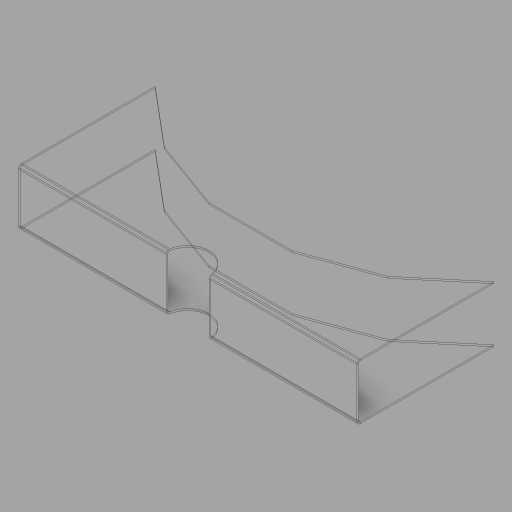
# Autodesk Inventor part: Halteblech
Saved by Autodesk Inventor 2023.2 (Build 272271000, 271)
## iProperties
Created: 2023-02-02
Part Number: Halteblech
Material: Generisch
Document SubType Name: Blech
Designer: Raoul Messerli
Density: 1 g/cm^3
Sheet Metal Rule: 3mm
Appearance: Vorgabe
Author: Raoul Messerli
Autodesk Inventor part; units mm, degrees
ref_plane "YZ Plane" through (0, 0, 0) normal (1, 0, 0) x (0, 1, 0)
ref_plane "XZ Plane" through (0, 0, 0) normal (0, 1, 0) x (-1, 0, 0)
ref_plane "XY Plane" through (0, 0, 0) normal (0, 0, 1) x (1, 0, 0)
sketch "Skizze1" plane through (0, 0, 0) normal (0, 0, 1) x (1, 0, 0)
  line L0 (300, -50) -> (-300, -50)
  line L1 (-300, -50) -> (-300, 50)
  line L2 (-300, 50) -> (300, 50)
  line L3 (300, 50) -> (300, -50)
  line L4 (300, -50) -> (-300, 50) construction
  line L5 (-300, -50) -> (300, 50) construction
  point P0 (0, 0)
  dimension "d0" = 600
  dimension "d1" = 100
  measures "d0" distance of L1.end L2.end
  measures "d1" distance of L0.end L1.end
extrude "Grobblech1" add sketch "Skizze1" along normal blind 3
sketch "Skizze2" plane through (300, 47, 3) normal (0, 1, 0) x (-1, 0, 0)
  line L0 (600, 0) -> (0, 0)
  line L1 (0, 0) -> (0, -250)
  line L2 (0, -250) -> (600, -250)
  line L3 (600, -250) -> (600, 0)
  constraints: 6 end point, 1 horizontal, 1 perpendicular, 1 vertical
edge flange "Lasche1" height 250 angle 90 thickness 3 bend radius 3 thickness toward (0, 1, 0) relief straight relief width 3 relief depth 1.5 edges at (0, 50, 0) wall of the first edge with corners at (-300, 47, 3) (300, 47, 3) (300, 47, -247) (-300, 47, -247)
bend "Biegung1"
corner "Ecke1"
sketch "Skizze3" plane through (-300, -47, 3) normal (0, -1, 0) x (1, 0, 0)
  line L0 (600, 0) -> (0, 0)
  line L1 (0, 0) -> (0, -250)
  line L2 (0, -250) -> (600, -250)
  line L3 (600, -250) -> (600, 0)
  constraints: 6 end point, 1 horizontal, 1 perpendicular, 1 vertical
edge flange "Lasche2" height 250 angle 90 thickness 3 bend radius 3 thickness toward (0, -1, 0) relief straight relief width 3 relief depth 1.5 edges at (0, -50, 0) wall of the first edge with corners at (300, -47, 3) (-300, -47, 3) (-300, -47, -247) (300, -47, -247)
bend "Biegung2"
corner "Ecke2"
sketch "Skizze4" plane through (0, 0, 0) normal (0, 1, 0) x (-1, 0, 0)
  line L0 (300, 3) -> (-300, 3) projected
  circle A0 centre (0, 3) radius 38.05
  point P0 (0, 0)
  dimension "d23" = 76.1
  constraints: 1 centre point, 1 midpoint
  measures "d23" diameter of A0
extrude "Extrusion1" cut sketch "Skizze4" along normal through all both and the other way through all
sketch "Skizze5" plane through (0, 0, 0) normal (0, 1, 0) x (-1, 0, 0)
  line L0 (-300, -3) -> (-300, -247) projected
  line L1 (-300, -239.3955) -> (-198.2712, -154.035)
  line L2 (-198.2712, -154.035) -> (-73.4825, -108.6156)
  line L3 (-73.4825, -108.6156) -> (73.4825, -108.6156)
  line L4 (73.4825, -108.6156) -> (198.2712, -154.035)
  line L5 (198.2712, -154.035) -> (300, -239.3955)
  line L6 (300, -3) -> (300, -247) projected
  line L7 (-300, -239.3955) -> (-300, -247)
  line L8 (-300, -247) -> (300, -247)
  line L9 (300, -247) -> (300, -239.3955)
  point P0 (0, 0)
  dimension "d26" = 160
  dimension "d27" = 160
  dimension "d28" = 160
  dimension "d29" = 160
  constraints: 16 end point, 3 equal length, 2 point on line, 1 collinear, 1 perpendicular
  measures "d26" angle of L3 L4
  measures "d27" angle of L5 L4
  measures "d28" angle of L3 L2
  measures "d29" angle of L1 L2
extrude "Extrusion2" cut sketch "Skizze5" along normal through all both and the other way through all
equation "\"d2\" = Stärke"
equation "\"d3\" = BreiteBiegungsfreistellung"
equation "\"d4\" = TiefeBiegungsfreistellung"
equation "\"d5\" = MinimalRest"
equation "\"d6\" = Übergangsradius"
equation "\"d9\" = Biegeradius"
equation "\"d10\" = GrößeEckenfreistellung"
equation "\"d11\" = Abstandsgröße"
equation "\"d12\" = JacobiRadiusGröße"
equation "\"d13\" = BreiteBiegungsfreistellung"
equation "\"d14\" = TiefeBiegungsfreistellung"
equation "\"d15\" = MinimalRest"
equation "\"d16\" = Übergangsradius"
equation "\"d19\" = Biegeradius"
equation "\"d20\" = GrößeEckenfreistellung"
equation "\"d21\" = Abstandsgröße"
equation "\"d22\" = JacobiRadiusGröße"
equation "\"Biegeradius\" = Stärke"
equation "\"BreiteBiegungsfreistellung\" = Stärke"
equation "\"TiefeBiegungsfreistellung\" = 0.5 * Stärke"
equation "\"GrößeEckenfreistellung\" = 4 * Stärke"
equation "\"MinimalRest\" = 2 * Stärke"
equation "\"Übergangsradius\" = Biegeradius"
equation "\"JacobiRadiusGröße\" = Biegeradius"
equation "\"Stärke\" = 3"
equation "\"Abstandsgröße\" = 3"
